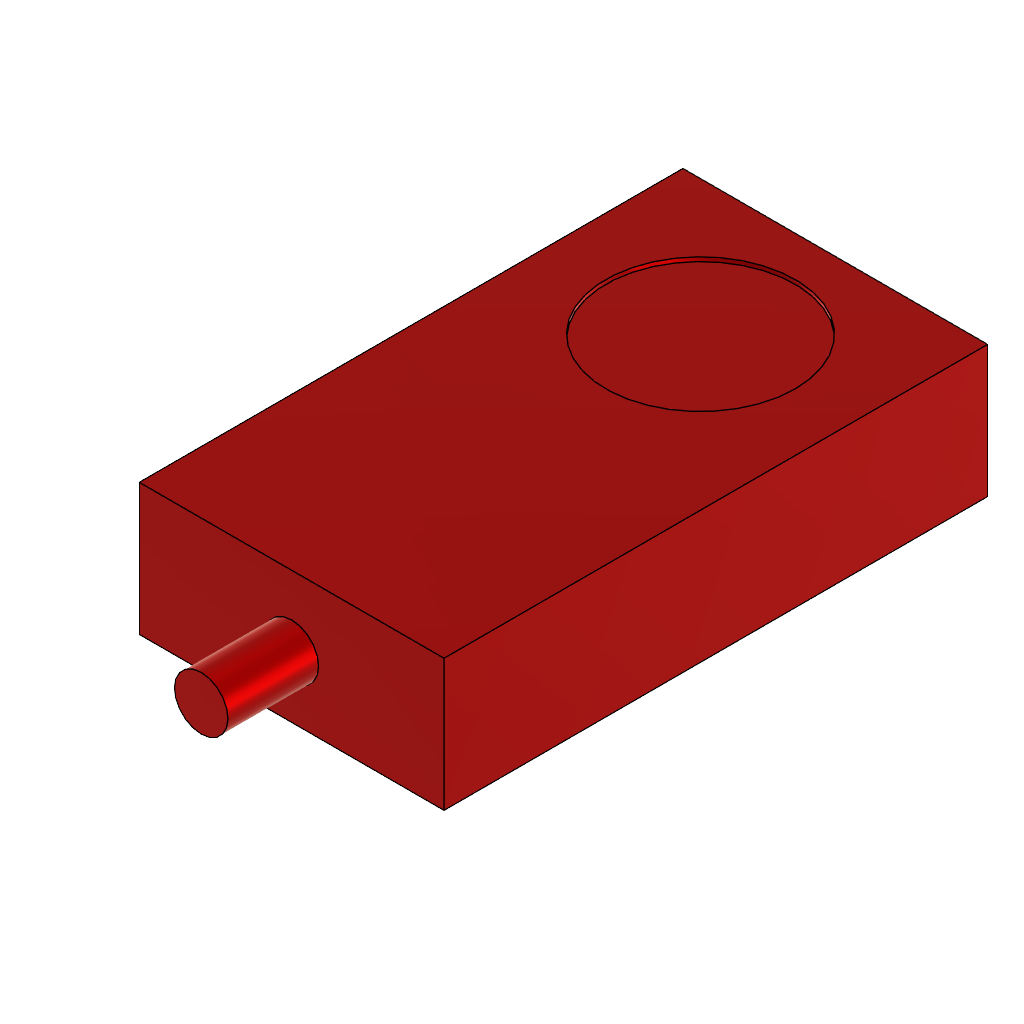
VTX_Foxeer_Reaper_Inf (Autodesk Fusion 360 design; units mm, degrees)
part number: 2026-09-23-14-11-19-425
Autodesk Fusion 360 part; units mm, degrees
sketch "Sketch1" plane through (0, 0, 0) normal (0, 0, 1) x (1, 0, 0)
  line L0 (-18.5, 33) -> (18.5, 33)
  line L1 (18.5, 33) -> (18.5, -33)
  line L2 (18.5, -33) -> (-18.5, -33)
  line L3 (-18.5, -33) -> (-18.5, 33)
  line L4 (-18.5, 33) -> (18.5, -33) construction
  line L5 (18.5, 33) -> (-18.5, -33) construction
  dimension "d1" = 37
  dimension "d2" = 66
  constraint horizontal L0
  constraint perpendicular L0 L1
  constraint parallel L0 L2
  constraint parallel L1 L3
  constraint coincident L4 origin
  constraint coincident L5 origin
  measures "d1" distance of L1.end L2.end
  measures "d2" distance of L0.end L1.end
extrude "Extrude1" add sketch "Sketch1" along normal blind 16 makes body 1
sketch "Sketch2" plane through (0, 0, 0) normal (0, 0, 1) x (1, 0, 0)
  line L0 (10, -10) -> (-10, -10) construction
  line L1 (-10, -10) -> (-10, 10) construction
  line L2 (-10, 10) -> (10, 10) construction
  line L3 (10, 10) -> (10, -10) construction
  line L4 (10, -10) -> (-10, 10) construction
  line L5 (-10, -10) -> (10, 10) construction
  circle A0 centre (10, 10) radius 1
  circle A1 centre (10, -10) radius 1
  circle A2 centre (-10, 10) radius 1
  circle A3 centre (-10, -10) radius 1
  dimension "d5" = 2
  dimension "d6" = 2
  dimension "d7" = 2
  dimension "d8" = 2
  constraint horizontal L0
  constraint perpendicular L0 L1
  constraint parallel L0 L2
  constraint parallel L1 L3
  constraint coincident L4 origin
  constraint coincident L5 origin
  constraint coincident L2.end L3.start
  constraint coincident L0.start L3.end
  constraint coincident L1.end L2.start
  constraint coincident L0.end L1.start
  measures "d5" diameter of A0
  measures "d6" diameter of A1
  measures "d7" diameter of A2
  measures "d8" diameter of A3
extrude "Extrude2" cut sketch "Sketch2" along normal blind 2.5 bodies 1
sketch "Sketch3" plane through (0, -33, 0) normal (0, -1, 0) x (1, 0, 0)
  line L0 (-18.5, 0) -> (18.5, 0)
  line L1 (18.5, 0) -> (18.5, 16)
  line L2 (18.5, 16) -> (-18.5, 16)
  line L3 (-18.5, 16) -> (-18.5, 0)
  circle A0 centre (0, 7.5245) radius 3.25
  dimension "d11" = 6.5
  measures "d11" diameter of A0
sketch "Sketch4" plane through (0, -33, 0) normal (0, -1, 0) x (1, 0, 0)
  line L0 (-18.5, 0) -> (18.5, 0)
  line L1 (18.5, 0) -> (18.5, 16)
  line L2 (18.5, 16) -> (-18.5, 16)
  line L3 (-18.5, 16) -> (-18.5, 0)
  circle A0 centre (0.0221, 7.5311) radius 3.25
  dimension "d12" = 6.5
  measures "d12" diameter of A0
extrude "Extrude3" add sketch "Sketch4" along normal blind 11 contours A0 bodies 1
sketch "Sketch5" plane through (0, 0, 16) normal (0, 0, 1) x (-1, 0, 0)
  line L0 (18.5, 33) -> (-18.5, 33)
  line L1 (-18.5, 33) -> (-18.5, -33)
  line L2 (-18.5, -33) -> (18.5, -33)
  line L3 (18.5, -33) -> (18.5, 33)
  circle A0 centre (0, -16.6341) radius 11.5
  dimension "d15" = 23
  measures "d15" diameter of A0
extrude "Extrude4" cut sketch "Sketch5" against normal blind 0.5 contours A0 bodies 1
sketch "Sketch6" plane through (-18.5, 0, 0) normal (-1, 0, 0) x (0, -1, 0)
  line L0 (-33, 0) -> (33, 0)
  line L1 (33, 0) -> (33, 16)
  line L2 (33, 16) -> (-33, 16)
  line L3 (-33, 16) -> (-33, 0)
  line L4 (-28, 6) -> (-21, 6)
  line L5 (-21, 6) -> (-21, 4)
  line L6 (-21, 4) -> (-28, 4)
  line L7 (-28, 4) -> (-28, 6)
  constraint horizontal L4
  constraint vertical L5
  constraint horizontal L6
  constraint vertical L7
extrude "Extrude5" add sketch "Sketch6" along normal blind 1.5 separate body contours L4 L5 L6 L7 makes body 2
sketch "Sketch7" plane through (0, 33, 0) normal (0, 1, 0) x (-1, 0, 0)
  line L0 (-18.5, 0) -> (18.5, 0)
  line L1 (18.5, 0) -> (18.5, 16)
  line L2 (18.5, 16) -> (-18.5, 16)
  line L3 (-18.5, 16) -> (-18.5, 0)
  line L4 (-5, 8) -> (5, 8)
  line L5 (5, 8) -> (5, 5)
  line L6 (5, 5) -> (-5, 5)
  line L7 (-5, 5) -> (-5, 8)
  constraint horizontal L4
  constraint vertical L5
  constraint horizontal L6
  constraint vertical L7
extrude "Extrude6" cut sketch "Sketch7" against normal blind 1.5 contours L4 L5 L6 L7 bodies 1
combine "Combine1" operation add target body 1 tool bodies 2
